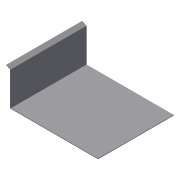
# Autodesk Inventor part: ToteBasin
Saved by Autodesk Inventor 2015 (Build 190159000, 159)
## iProperties
Created: 2015-03-06
Part Number: ToteBasin
Material: Generic
Document SubType Name: Modeling
Designer: Jaden
Density: 1 g/cm^3
Appearance: Default
Author: Jaden
Autodesk Inventor part; units mm, degrees
ref_plane "YZ Plane" through (0, 0, 0) normal (1, 0, 0) x (0, 1, 0)
ref_plane "XZ Plane" through (0, 0, 0) normal (0, 1, 0) x (-1, 0, 0)
ref_plane "XY Plane" through (0, 0, 0) normal (0, 0, 1) x (1, 0, 0)
sketch "Sketch1" plane through (0, 0, 0) normal (0, 0, 1) x (1, 0, 0)
  line L0 (0, 0) -> (-23.2949, 10.1247)
  line L1 (0, 0) -> (25.4, 0) construction
  line L2 (-23.2949, 10.1247) -> (-24.5605, 7.2128)
  line L3 (-24.5605, 7.2128) -> (-4.1774, -1.6463)
  line L4 (0, -74.676) -> (304.8, -74.676)
  line L5 (304.8, -74.676) -> (304.8, -77.851)
  line L6 (304.8, -77.851) -> (-4.1774, -77.8463)
  line L7 (-4.1774, -1.6463) -> (-4.1774, -179.4463)
  line L8 (-4.1774, -1.6463) -> (173.6226, -1.6463) construction
  line L9 (0, 0) -> (0, -176.276)
  line L10 (0, 0) -> (176.276, 0) construction
  line L11 (0, -176.276) -> (457.2, -176.276)
  line L12 (457.2, -176.276) -> (457.2, -179.451)
  line L13 (457.2, -179.451) -> (-4.1774, -179.4463)
  dimension "d0" = 25.4
  dimension "d1" = 156.509
  dimension "d2" = 3.175
  dimension "d3" = 90
  dimension "d4" = 22.225
  dimension "d5" = 90
  dimension "d8" = 304.8
  dimension "d10" = 3.175
  dimension "d13" = 177.8
  dimension "d14" = 90
  dimension "d15" = 176.276
  dimension "d16" = 90
  dimension "d17" = 457.2
  dimension "d18" = 90
  dimension "d19" = 3.175
  constraints: 28 end point, 4 perpendicular, 3 equal length, 3 horizontal, 3 vertical
  measures "d0" distance of L0.start L0.end
  measures "d1" angle of L1 L0
  measures "d2" distance of L0.end L2.end
  measures "d3" angle of L2 L0
  measures "d4" distance of L2.end L3.end
  measures "d5" angle of L3 L2
  measures "d8" distance of L4.start L4.end
  measures "d10" distance of L4.end L5.end
  measures "d13" distance of L3.end L7.end
  measures "d14" angle of L7 L8
  measures "d15" distance of L0.start L9.end
  measures "d16" angle of L9 L10
  measures "d17" distance of L9.end L11.end
  measures "d18" angle of L11 L9
  measures "d19" distance of L11.end L12.end
extrude "Extrusion2" add sketch "Sketch1" along normal blind 396.875 contours L9 L6 L7 L3 L2 L0 | L9 L11 L12 L13 L7 L6
body "Solid2"
